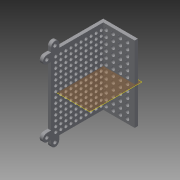
# Autodesk Inventor part: BattCradke
Saved by Autodesk Inventor 2014 SP1 (Build 180222100, 222)
## iProperties
Created: 2017-01-20
Part Number: BattCradke
Material: Generic
Document SubType Name: Modeling
Designer: danielsikar
Density: 1 g/cm^3
Appearance: Default
Author: danielsikar
Autodesk Inventor part; units mm, degrees
ref_plane "YZ Plane" through (0, 0, 0) normal (1, 0, 0) x (0, 1, 0)
ref_plane "XZ Plane" through (0, 0, 0) normal (0, 1, 0) x (-1, 0, 0)
ref_plane "XY Plane" through (0, 0, 0) normal (0, 0, 1) x (1, 0, 0)
sketch "Sketch1" plane through (0, 0, 0) normal (0, 0, 1) x (1, 0, 0)
  line L0 (21.1051, -223.4207) -> (21.1051, -163.9207) projected
  line L1 (21.1051, -163.9207) -> (39.6051, -163.9207) projected
  line L2 (39.6051, -223.4207) -> (39.6051, -163.9207) projected
  line L3 (21.1051, -223.4207) -> (39.6051, -223.4207) projected
  line L4 (16.1051, -220.9207) -> (16.1051, -163.9207) projected
  line L5 (5.6051, -220.9207) -> (16.1051, -220.9207) projected
  line L6 (5.6051, -220.9207) -> (5.6051, -163.9207) projected
  line L7 (5.6051, -163.9207) -> (16.1051, -163.9207) projected
  line L8 (39.6051, -223.4207) -> (5.6051, -223.4207)
  line L9 (5.6051, -223.4207) -> (5.6051, -163.9207)
  line L10 (5.6051, -163.9207) -> (39.6051, -163.9207)
  line L11 (39.6051, -163.9207) -> (39.6051, -223.4207)
  line L12 (39.9051, -223.7207) -> (5.3051, -223.7207)
  line L13 (5.3051, -223.7207) -> (5.3051, -163.6207)
  line L14 (5.3051, -163.6207) -> (39.9051, -163.6207)
  line L15 (39.9051, -163.6207) -> (39.9051, -223.7207)
  line L16 (43.9051, -227.7207) -> (1.3051, -227.7207)
  line L17 (1.3051, -227.7207) -> (1.3051, -159.6207)
  line L18 (1.3051, -159.6207) -> (43.9051, -159.6207)
  line L19 (43.9051, -159.6207) -> (43.9051, -227.7207)
  point P0 (0, 0)
  dimension "d0" = 0.3
  dimension "d1" = 4
  constraints: 24 end point, 6 parallel, 3 perpendicular, 1 horizontal, 6 other
  measures "d0" distance between parallel lines of L15 L2
  measures "d1" distance between parallel lines of L19 L15
extrude "Extrusion1" add sketch "Sketch1" against normal blind 93 contours L16 L17 L18 L19
sketch "Sketch3" plane through (1.3051, -159.6207, 0) normal (0, 1, 0) x (1, 0, 0)
  line L0 (0, 0) -> (42.6, 0) projected
  line L1 (0, 0) -> (0, 93) projected
  circle A0 centre (7, 6) radius 2.5
  point P0 (-1.3051, 0)
  dimension "d4" = 5
  dimension "d5" = 6
  dimension "d6" = 7
  constraints: 1 centre point
  measures "d4" diameter of A0
  measures "d5" distance from line of A0.centre L0
  measures "d6" distance from line of A0.centre L1
extrude "Extrusion2" cut sketch "Sketch3" against normal blind 20
pattern_linear "Rectangular Pattern1" count 12 spacing 7.4 along (0, 0, -1) count 4 spacing 8.8 along (1, 0, 0) of "Extrusion2"
sketch "Sketch4" plane through (1.3051, -227.7207, 0) normal (-1, 0, 0) x (0, 0, 1)
  line L0 (0, 0) -> (0, 68.1) projected
  line L1 (0, 0) -> (-93, 0) projected
  circle A0 centre (-7, 6) radius 2
  point P0 (0, 227.7207)
  dimension "d15" = 4
  dimension "d16" = 6
  dimension "d17" = 7
  constraints: 1 centre point
  measures "d15" diameter of A0
  measures "d16" distance from line of L1 A0.centre
  measures "d17" distance from line of L0 A0.centre
extrude "Extrusion3" cut sketch "Sketch4" against normal blind 20
pattern_linear "Rectangular Pattern2" count 14 spacing 6.2 along (0, 0, -1) count 10 spacing 6.2 along (0, 1, 0) of "Extrusion3"
sketch "Sketch5" plane through (0, 0, 0) normal (0, 0, 1) x (1, 0, 0)
  line L0 (39.9051, -163.6207) -> (39.9051, -223.7207) projected
  line L1 (39.9051, -223.7207) -> (5.3051, -223.7207) projected
  line L2 (5.3051, -223.7207) -> (5.3051, -163.6207) projected
  line L3 (5.3051, -163.6207) -> (39.9051, -163.6207) projected
  line L4 (43.9051, -227.7207) -> (1.3051, -227.7207) projected
  line L5 (43.9051, -159.6207) -> (43.9051, -227.7207) projected
  line L6 (5.3051, -227.7207) -> (43.9051, -227.7207)
  line L7 (43.9051, -227.7207) -> (43.9051, -163.6207)
  line L8 (43.9051, -163.6207) -> (5.3051, -163.6207)
  line L9 (5.3051, -163.6207) -> (5.3051, -227.7207)
  point P0 (0, 0)
  constraints: 8 end point, 2 parallel, 2 point on line, 1 horizontal, 1 perpendicular
extrude "Extrusion4" cut sketch "Sketch5" against normal through all contours L8 L5 L4 L9 L1 L0
sketch "Sketch6" plane through (1.3051, -227.7207, 0) normal (0, -1, 0) x (1, 0, 0)
  line L0 (4, -93) -> (4, 0) projected
  line L1 (0, 0) -> (4, 0)
  line L2 (4, 0) -> (4, -10)
  line L3 (4, -10) -> (0, -10)
  line L4 (0, -10) -> (0, 0)
  point P0 (-1.3051, 0)
  dimension "d28" = 10
  constraints: 8 end point, 2 parallel, 1 horizontal, 1 perpendicular, 1 point on line
  measures "d28" distance of L1.end L2.end
extrude "Extrusion5" add sketch "Sketch6" along normal blind 10
sketch "Sketch7" plane through (5.3051, -227.7207, -93) normal (1, 0, 0) x (0, 0, -1)
  circle A0 centre (-88, -5) radius 2.15
  point P0 (-93, 227.7207)
  dimension "d31" = 4.3
  constraints: 1 centre point
  measures "d31" diameter of A0
extrude "Extrusion6" cut sketch "Sketch7" against normal blind 10
sketch "Sketch8" plane through (0, 0, 0) normal (0, 0, 1) x (1, 0, 0)
  line L0 (5.3051, -237.7207) -> (5.3051, -163.6207) projected
  line L1 (1.3051, -159.6207) -> (1.3051, -237.7207) projected
  line L2 (5.3051, -237.7207) -> (1.3051, -237.7207) projected
  line L3 (5.3051, -227.7207) -> (1.3051, -227.7207)
  line L4 (1.3051, -227.7207) -> (1.3051, -217.7207)
  line L5 (1.3051, -217.7207) -> (5.3051, -217.7207)
  line L6 (5.3051, -217.7207) -> (5.3051, -227.7207)
  point P0 (0, 0)
  dimension "d34" = 10
  dimension "d35" = 10
  constraints: 8 end point, 2 parallel, 2 point on line, 1 horizontal, 1 perpendicular
  measures "d34" distance of L3.end L4.end
  measures "d35" distance between parallel lines of L3 L2
extrude "Extrusion7" add sketch "Sketch8" along normal blind 10 contours L3 L1 L5 L0
sketch "Sketch10" plane through (5.3051, -227.7207, -93) normal (1, 0, 0) x (0, 0, -1)
  circle A0 centre (-98, 5) radius 2.15
  point P0 (-93, 227.7207)
  dimension "d38" = 4.3
  constraints: 1 centre point
  measures "d38" diameter of A0
extrude "Extrusion8" cut sketch "Sketch10" against normal blind 10
fillet "Fillet1" radius 5 4 edges at (3.3051, -237.7207, -10) (3.3051, -237.7207, 0) (3.3051, -227.7207, 10) (3.3051, -217.7207, 10)
ref_plane "Work Plane1" through (0, 0, -46.5) normal (0, 0, 1) x (1, 0, 0)
mirror "Mirror2" about plane through (0, 0, -46.5) normal (0, 0, 1) of "Extrusion5", "Extrusion6", "Extrusion7", "Extrusion8", "Fillet1"
body "Solid1"
